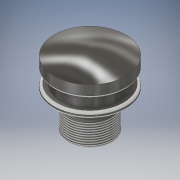
# Autodesk Inventor part: ventplug
Saved by Autodesk Inventor 2017 (Build 210142000, 142)
## iProperties
Created: 2020-01-12
Part Number: ventplug
Material: Generic
Document SubType Name: Modeling
Designer: Admin
Density: 1 g/cm^3
Appearance: Default
Mass: 0.380128 g
Surface Area: 4.05583 cm^2
Volume: 0.380128 cm^3
Author: Admin
Autodesk Inventor part; units mm, degrees
ref_plane "YZ Plane" through (0, 0, 0) normal (1, 0, 0) x (0, 1, 0)
ref_plane "XZ Plane" through (0, 0, 0) normal (0, 1, 0) x (-1, 0, 0)
ref_plane "XY Plane" through (0, 0, 0) normal (0, 0, 1) x (1, 0, 0)
sketch "Sketch1" plane through (0, 0, 0) normal (0, 1, 0) x (-1, 0, 0)
  circle A0 centre (0, 0) radius 2.8956
  dimension "d0" = 5.7912
  constraints: 1 centre point, 1 coincident
  measures "d0" diameter of A0
extrude "Extrusion1" add sketch "Sketch1" against normal blind 4.7625
sketch "Sketch4" plane through (0, 0, 0) normal (0, 1, 0) x (1, 0, 0)
  circle A0 centre (0, 0) radius 2.5422
  circle A1 centre (0, 0) radius 2.8956
  dimension "d4" = 5.7912
  dimension "d5" = 5.0843
  constraints: 2 centre point, 2 coincident
  measures "d4" diameter of A1
  measures "d5" diameter of A0
extrude "Extrusion2" cut sketch "Sketch4" against normal blind 1.5875
sketch "Sketch5" plane through (0, 0, 0) normal (0, 1, 0) x (1, 0, 0)
  circle A0 centre (0, 0) radius 4.7625
  dimension "d8" = 9.525
  constraints: 1 centre point, 1 coincident
  measures "d8" diameter of A0
extrude "Extrusion3" add sketch "Sketch5" along normal blind 0.7937
sketch "Sketch6" plane through (0, 0.7937, 0) normal (0, 1, 0) x (1, 0, 0)
  circle A0 centre (0, 0) radius 3.9688
  dimension "d11" = 7.9375
  constraints: 1 centre point, 1 coincident
  measures "d11" diameter of A0
extrude "Extrusion4" add sketch "Sketch6" along normal blind 1.5875
sketch "Sketch7" plane through (0, 2.3812, 0) normal (0, 1, 0) x (1, 0, 0)
  circle A0 centre (0, 0) radius 4.7625
  dimension "d14" = 9.525
  constraints: 1 centre point, 1 coincident
  measures "d14" diameter of A0
extrude "Extrusion5" add sketch "Sketch7" along normal blind 1.5875
sketch "Sketch8" plane through (0, 0, 0) normal (0, 0, 1) x (1, 0, 0)
  line L0 (4.7625, 3.9688) -> (-4.7625, 3.9688) projected
  line L1 (0, 3.9688) -> (4.7625, 3.9688)
  line L2 (0, 3.9688) -> (0, 4.7625)
  arc A0 (4.7625, 3.9688) -> (0, 4.7625) centre (-0.7253, -14.2737) ccw
  line L3 (0, -18.1112) -> (0, 8.7515) projected
  point P0 (0, 0)
  dimension "d17" = 0.7937
  dimension "d18" = 19.05
  constraints: 4 end point, 2 point on circle, 1 centre point, 1 collinear, 1 midpoint, 1 perpendicular
  measures "d17" distance of L1.start L2.end
  measures "d18" radius of A0
revolve "Revolution1" add sketch "Sketch8" angle 360 about axis through (0, -10, 0) along (0, 1, 0)
sketch "Sketch9" plane through (0, -4.7625, 0) normal (0, -1, 0) x (1, 0, 0)
  point P0 (0, 0)
  point P1 (0, 0)
  constraints: 1 coincident
hole "Hole1" at (0, -4.7625, 0) direction (0, 1, 0) diameter 1.1811 depth 7.1437 tip angle 118
thread "Thread1" size "00-90 NS" class "2A" standard "ANSI Unified Screw Threads" full length
fillet "Fillet1" radius 0.3175 4 edges at (-4.7625, 0, 0) (-4.7625, 0.7937, 0) (-4.7625, 2.3812, 0) (2.8956, -4.7625, 0)
body "Solid1"
